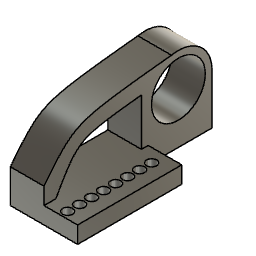
tensor v5 v2 (Autodesk Fusion 360 design; units mm, degrees)
Autodesk Fusion 360 part; units mm, degrees
note: some values were not read from the file. Set by a fixed rule: which sketch regions a step uses.
sketch "Sketch1" plane through (0, 0, 0) normal (0, 0, 1) x (1, 0, 0)
  line L0 (0, 0) -> (20, 0)
  line L1 (20, 0) -> (20, 50)
  line L2 (20, 50) -> (0, 50)
  line L3 (0, 50) -> (0, 0)
  dimension "d1" = 50
  constraint horizontal L0
  constraint vertical L1
  constraint horizontal L2
  constraint vertical L3
  constraint coincident L0.start L3.end
  measures "d1" distance of L0.start L2.end
extrude "Extrude1" add sketch "Sketch1" along normal blind 30
sketch "Sketch2" plane through (0, 0, 0) normal (0, -1, 0) x (1, 0, 0)
  line L0 (0, 0) -> (20, 0)
  line L1 (20, 0) -> (20, 30)
  line L2 (20, 30) -> (0, 30)
  line L3 (0, 30) -> (0, 0)
  line L4 (0, 30) -> (10, 30)
  line L5 (20, 0) -> (20, 5)
  line L6 (20, 5) -> (10, 5)
  line L7 (10, 5) -> (10, 30)
  dimension "d4" = 5
  constraint coincident L2.end L3.start
  constraint midpoint L2 L4.end
  constraint coincident L0.end L1.start
  constraint perpendicular L0 L5
  constraint perpendicular L1 L6
  constraint perpendicular L2 L7
  measures "d4" distance of L0.end L5.end
extrude "Extrude2" cut sketch "Sketch2" against normal blind 70 contours L1 L2 L6 L7
sketch "Sketch3" plane through (0, 0, 0) normal (-1, 0, 0) x (0, -1, 0)
  line L0 (-50, 0) -> (0, 0)
  line L1 (0, 0) -> (0, 30)
  line L2 (0, 30) -> (-50, 30)
  line L3 (-50, 30) -> (-50, 0)
  line L4 (-50, 15) -> (-40, 15)
  line L5 (-40, 15) -> (-40, 30)
  circle A0 centre (-40, 15) radius 8
  dimension "d7" = 16
  constraint midpoint L3 L4.start
  constraint perpendicular L3 L4
  constraint coincident L2 L5.end
  constraint perpendicular L2 L5
  constraint coincident L4.end L5.start
  measures "d7" diameter of A0
extrude "Extrude3" cut sketch "Sketch3" against normal blind 15 contours L4 L5 A0 | L4 L5 A0
sketch "Sketch4" plane through (0, 0, 5) normal (0, 0, 1) x (-1, 0, 0)
  line L0 (-20, -50) -> (-10, -50)
  line L1 (-10, -50) -> (-10, 0)
  line L2 (-10, 0) -> (-20, 0)
  line L3 (-20, 0) -> (-20, -50)
  circle A0 centre (-15, -45) radius 0.25
  line L4 (-10, -30) -> (-20, -30)
  circle A1 centre (-15, -27.0301) radius 1.5
  circle A2 centre (-15, -23.4587) radius 1.5
  circle A3 centre (-15, -19.8873) radius 1.5
  circle A4 centre (-15, -16.3158) radius 1.5
  circle A5 centre (-15, -12.7444) radius 1.5
  circle A6 centre (-15, -9.173) radius 1.5
  circle A7 centre (-15, -5.6015) radius 1.5
  circle A8 centre (-15, -2.0301) radius 1.5
  dimension "d11" = 3
  dimension "d14" = 0
  dimension "d15" = 25
  constraint coincident L1 L4.start
  constraint coincident L3 L4.end
  constraint perpendicular L3 L4
  measures "d11" diameter of A1
extrude "Extrude4" cut sketch "Sketch4" against normal blind 15 contours A1 | A2 | A3 | A4 | A5 | A6 | A7 | A8
sketch "Sketch5" plane through (0, 0, 0) normal (-1, 0, 0) x (0, -1, 0)
  circle A0 centre (-40, 15) radius 8
  line L0 (-50, 0) -> (0, 0)
  line L1 (0, 0) -> (0, 30)
  line L2 (0, 30) -> (-50, 30)
  line L3 (-50, 30) -> (-50, 0)
  circle A1 centre (-40, 15) radius 10
  spline S0 degree 2 poles (-40, 25) (-9.0379, 21.8056) (0, 10) knots 0 0 0 4.447549 4.447549 4.447549 weights 1 3 1
  constraint concentric A0 A1
  constraint coincident L1 S0.end
  constraint coincident A1 S0.start
extrude "Extrude5" cut sketch "Sketch5" against normal blind 60 contours L1 L2 L3 A1 S0
sketch "Sketch6" plane through (0, 0, 0) normal (-1, 0, 0) x (0, -1, 0)
  arc A0 (-37.945, 24.7866) -> (-50, 15) centre (-40, 15) ccw
  line L0 (-50, 15) -> (-50, 0)
  line L1 (-50, 0) -> (0, 0)
  line L2 (0, 0) -> (0, 10)
  spline S0 degree 2 poles (0, 10) (-9.0024, 21.7593) (-37.945, 24.7866) knots -4.447549 -4.447549 -4.447549 -0.051947 -0.051947 -0.051947 weights 1 2.97664 1.046174
  circle A1 centre (-40, 15) radius 8
  line L3 (-3, 4) -> (-4, 4)
  line L4 (-4, 4) -> (-29, 4)
  line L5 (-29, 4) -> (-29, 19)
  spline S1 degree 2 poles (-29, 19) (-10, 17) (-3, 4) knots 0 0 0 3.222354 3.222354 3.222354 weights 1 3 1
  line L6 (-3.5416, 5) -> (-29, 5)
  constraint horizontal L3
  constraint parallel L3 L4
  constraint perpendicular L4 L5
  constraint coincident S1 L6.start
  constraint coincident L5 L6.end
  constraint perpendicular L5 L6
extrude "Extrude6" cut sketch "Sketch6" against normal blind 16 contours L5 S1 L6
sketch "Sketch7" plane through (0, 0, 5) normal (0, 0, 1) x (-1, 0, 0)
  circle A0 centre (-15, -9.173) radius 1.5
  circle A1 centre (-15, -5.6015) radius 1.5
  circle A2 centre (-15, -12.7444) radius 1.5
  circle A3 centre (-15, -16.3158) radius 1.5
  line L0 (-10, -3.5416) -> (-10, 0)
  line L1 (-10, 0) -> (-20, 0)
  line L2 (-20, 0) -> (-20, -50)
  line L3 (-20, -50) -> (-10, -50)
  line L4 (-10, -50) -> (-10, -29)
  line L5 (-10, -29) -> (0, -29)
  line L6 (0, -29) -> (0, -3.5416)
  line L7 (0, -3.5416) -> (-10, -3.5416)
  circle A4 centre (-15, -19.8873) radius 1.5
  circle A5 centre (-15, -27.0301) radius 1.5
  circle A6 centre (-15, -23.4587) radius 1.5
  circle A7 centre (-15, -2.0301) radius 1.5
  line L8 (-10, -50) -> (-10, -31)
  line L9 (-20, -31) -> (-10, -31)
  line L10 (-20, -31) -> (-20, -50)
  line L11 (-10, -50) -> (-20, -50)
  constraint coincident L3.end L4.start
  constraint coincident L4 L8.end
  constraint perpendicular L3 L8
  constraint coincident L2 L9.start
  constraint perpendicular L8 L9
  constraint coincident L2.end L3.start
extrude "Extrude7" cut sketch "Sketch7" against normal blind 15 contours L2 L3 L4 L8 L9 L10 L11
